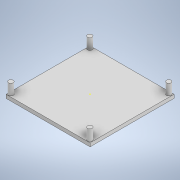
# Autodesk Inventor part: Camera Bottom
Saved by Autodesk Inventor 2020 (Build 240168000, 168)
## iProperties
Created: 2019-07-20
Part Number: Camera Bottom
Material: Generic
Document SubType Name: Modeling
Designer: Paul
Density: 1 g/cm^3
Appearance: Default
Author: Paul
Autodesk Inventor part; units mm, degrees
ref_plane "YZ Plane" through (0, 0, 0) normal (1, 0, 0) x (0, 1, 0)
ref_plane "XZ Plane" through (0, 0, 0) normal (0, 1, 0) x (-1, 0, 0)
ref_plane "XY Plane" through (0, 0, 0) normal (0, 0, 1) x (1, 0, 0)
sketch "Sketch1" plane through (0, 0, 0) normal (0, 1, 0) x (-1, 0, 0)
  line L0 (19, 19) -> (-19, 19)
  line L1 (-19, 19) -> (-19, -19)
  line L2 (-19, -19) -> (19, -19)
  line L3 (19, -19) -> (19, 19)
  dimension "d0" = 38
  dimension "d1" = 38
  constraints: 8 end point, 2 parallel, 1 horizontal, 1 perpendicular
  measures "d0" distance of L2.end L1.end
  measures "d1" distance of L1.end L0.end
extrude "Extrusion1" add sketch "Sketch1" along normal blind 1.6
sketch "Sketch2" plane through (0, 1.6, 0) normal (0, 1, 0) x (1, 0, 0)
  line L0 (19, -19) -> (19, 19) projected
  circle A0 centre (17.7429, 17.8888) radius 1.05
  circle A1 centre (17.7429, -17.8399) radius 1.05
  circle A2 centre (-17.9859, -17.8399) radius 1.05
  circle A3 centre (-17.9859, 17.8888) radius 1.05
  point P0 (0, 0)
  dimension "d7" = 2.1
  dimension "d8" = 2.1
  dimension "d9" = 2.1
  dimension "d10" = 2.1
  constraints: 4 centre point
  measures "d7" diameter of A0
  measures "d8" diameter of A1
  measures "d9" diameter of A2
  measures "d10" diameter of A3
extrude "Extrusion2" add sketch "Sketch2" along normal blind 4.95
sketch "Sketch3" plane through (0, 1.6, 0) normal (0, 1, 0) x (1, 0, 0)
  point P0 (0, 0)
body "Solid1"
